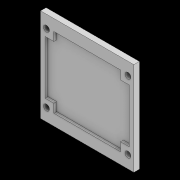
# Autodesk Inventor part: fan_controller_case_bottom
Saved by Autodesk Inventor 2022 (Build 260153000, 153)
## iProperties
Created: 2022-10-14
Part Number: fan_controller_case_bottom
Material: 一般
Document SubType Name: Modeling
Designer: numai
Density: 1 g/cm^3
Appearance: 既定
Author: numai
Autodesk Inventor part; units mm, degrees
ref_plane "YZ Plane" through (0, 0, 0) normal (1, 0, 0) x (0, 1, 0)
ref_plane "XZ Plane" through (0, 0, 0) normal (0, 1, 0) x (-1, 0, 0)
ref_plane "XY Plane" through (0, 0, 0) normal (0, 0, 1) x (1, 0, 0)
sketch "スケッチ1" plane through (0, 0, 0) normal (0, 0, 1) x (1, 0, 0)
  line L0 (-25.3, 21.7) -> (25.3, 21.7)
  line L1 (25.3, 21.7) -> (25.3, -21.7)
  line L2 (25.3, -21.7) -> (-25.3, -21.7)
  line L3 (-25.3, -21.7) -> (-25.3, 21.7)
  circle A0 centre (-22.1, 18.5) radius 1.6
  circle A1 centre (22.1, 18.5) radius 1.6
  circle A2 centre (22.1, -18.5) radius 1.6
  circle A3 centre (-22.1, -18.5) radius 1.6
  line L4 (-18.1, 19.2) -> (-18.1, 14.5)
  line L5 (-18.1, 14.5) -> (-22.8, 14.5)
  line L6 (-22.8, 14.5) -> (-22.8, -14.5)
  line L7 (-22.8, -14.5) -> (-18.1, -14.5)
  line L8 (-18.1, -14.5) -> (-18.1, -19.2)
  line L9 (-18.1, -19.2) -> (18.1, -19.2)
  line L10 (18.1, -19.2) -> (18.1, -14.5)
  line L11 (18.1, -14.5) -> (22.8, -14.5)
  line L12 (22.8, -14.5) -> (22.8, 14.5)
  line L13 (22.8, 14.5) -> (18.1, 14.5)
  line L14 (18.1, 14.5) -> (18.1, 19.2)
  line L15 (18.1, 19.2) -> (-18.1, 19.2)
  point P0 (0, 0)
  point P1 (0, 21.7)
  point P2 (-25.3, 0)
  dimension "d0" = 50.6
  dimension "d1" = 43.4
  dimension "d2" = 3.2
  dimension "d3" = 44.2
  dimension "d4" = 37
  dimension "d5" = 22.1
  dimension "d6" = 18.5
  dimension "d7" = 2.5
  dimension "d8" = 2.5
  dimension "d9" = 2.5
  dimension "d10" = 2.5
  dimension "d11" = 4
  dimension "d12" = 4
  dimension "d13" = 4
  dimension "d14" = 4
  dimension "d15" = 4
  constraints: 32 end point, 8 perpendicular, 6 point on line, 4 centre point, 3 equal radius, 3 horizontal alignment, 3 parallel, 3 vertical alignment, 2 midpoint, 1 horizontal, 1 vertical
  measures "d0" distance of L0.start L0.end
  measures "d1" distance of L0.end L1.end
  measures "d2" diameter of A0
  measures "d3" distance of A1.centre A0.centre
  measures "d4" distance of A3.centre A0.centre
  measures "d5" horizontal distance of point (0, 0) A1.centre
  measures "d6" vertical distance of point (0, 0) A0.centre
  measures "d7" distance between parallel lines of L0 L15
  measures "d8" distance between parallel lines of L3 L6
  measures "d9" distance between parallel lines of L2 L9
  measures "d10" distance between parallel lines of L1 L12
  measures "d11" distance from line of L5 A0.centre
  measures "d12" distance from line of L4 A0.centre
  measures "d13" distance from line of L14 A1.centre
  measures "d14" distance from line of A3.centre L7
  measures "d15" distance from line of L10 A2.centre
extrude "押し出し1" add sketch "スケッチ1" along normal blind 1.5
sketch "スケッチ2" plane through (0, 0, 0) normal (0, 0, -1) x (-1, 0, 0)
  line L0 (-25.3, 21.7) -> (25.3, 21.7) projected
  line L1 (-25.3, -21.7) -> (-25.3, 21.7) projected
  circle A0 centre (-22.1, 18.5) radius 1.6 projected
  line L2 (25.3, -21.7) -> (-25.3, -21.7) projected
  circle A1 centre (-22.1, -18.5) radius 1.6 projected
  circle A2 centre (22.1, -18.5) radius 1.6 projected
  line L3 (25.3, 21.7) -> (25.3, -21.7) projected
  circle A3 centre (22.1, 18.5) radius 1.6 projected
  point P0 (0, 0)
extrude "押し出し2" add sketch "スケッチ2" along normal blind 1.5
sketch "スケッチ3" plane through (-25.3, 21.7, 1.5) normal (0, 1, 0) x (1, 0, 0)
  line L0 (0, 3) -> (0, 0) projected
  line L1 (50.6, 0) -> (0, 0) projected
  line L2 (50.6, 3) -> (50.6, 0) projected
  line L3 (0, 3) -> (50.6, 3) projected
  point P0 (25.3, 1.5)
extrude "押し出し3" add sketch "スケッチ3" along normal blind 3.6
sketch "スケッチ4" plane through (-25.3, -21.7, 1.5) normal (0, -1, 0) x (1, 0, 0)
  line L0 (50.6, -3) -> (50.6, 0) projected
  line L1 (0, 0) -> (50.6, 0) projected
  line L2 (0, 0) -> (0, -3) projected
  line L3 (50.6, -3) -> (0, -3) projected
  point P0 (25.3, -1.5)
extrude "押し出し4" add sketch "スケッチ4" along normal blind 3.6
equation "\"d5\" = 0.5 * d3"
equation "\"d6\" = 0.5 * d4"
equation "\"d8\" = d7"
equation "\"d9\" = d7"
equation "\"d10\" = d7"
equation "\"d12\" = d11"
equation "\"d13\" = d11"
equation "\"d14\" = d11"
equation "\"d15\" = d11"
